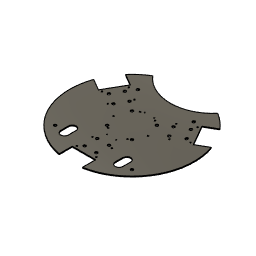
Plate_Mid+Desenho (Autodesk Fusion 360 archive; units mm, degrees)
design "Plate_Mid"
Autodesk Fusion 360 part; units mm, degrees
sketch "Esboço1" plane through (0, 0, 0) normal (0, 0, 1) x (1, 0, 0)
  circle A0 centre (0, 0) radius 240
  line L0 (48, -48) -> (-48, -48)
  line L1 (-48, -48) -> (-48, 48)
  line L2 (-48, 48) -> (48, 48)
  line L3 (48, 48) -> (48, -48)
  line L4 (48, -48) -> (-48, 48) construction
  line L5 (-48, -48) -> (48, 48) construction
  circle A1 centre (-48, 48) radius 5
  circle A2 centre (-48, -48) radius 5
  circle A3 centre (48, 48) radius 5
  circle A4 centre (48, -48) radius 5
  line L6 (105, -110) -> (105, -170)
  line L7 (90, -125) -> (90, -155)
  line L8 (120, -125) -> (120, -155)
  arc A5 (120, -125) -> (90, -125) centre (105, -125) ccw
  arc A6 (90, -155) -> (120, -155) centre (105, -155) ccw
  circle A7 centre (148, -148) radius 5
  line L9 (-125, 204.878) -> (125, 204.878)
  circle A8 centre (0, 311.043) radius 164
  circle A9 centre (107.5, 130.5) radius 5
  line L10 (-40, 115) -> (40, 115)
  line L11 (-40, 115) -> (-40, 151.9958)
  line L12 (40, 115) -> (40, 151.9958)
  line L13 (0, 1.75) -> (0, 22.5)
  line L14 (-120, -125) -> (-120, -155)
  arc A10 (-90, -125) -> (-120, -125) centre (-105, -125) ccw
  line L15 (-90, -125) -> (-90, -155)
  arc A11 (-120, -155) -> (-90, -155) centre (-105, -155) ccw
  circle A12 centre (-148, -148) radius 5
  circle A13 centre (-107.5, 130.5) radius 5
  line L16 (-45, -185) -> (45, -185)
  line L17 (45, -185) -> (45, -240)
  line L18 (45, -240) -> (-45, -240)
  line L19 (-45, -240) -> (-45, -185)
  line L20 (0, -185) -> (0, -175)
  line L21 (-37.5, -175) -> (37.5, -175)
  circle A14 centre (-37.5, -175) radius 2.5
  circle A15 centre (37.5, -175) radius 2.5
  circle A16 centre (37.5, -115) radius 2.5
  circle A17 centre (37.5, -55) radius 2.5
  circle A18 centre (-37.5, -115) radius 2.5
  circle A19 centre (-37.5, -55) radius 2.5
  circle A20 centre (132.8044, 119.976) radius 2.5
  line L22 (230.3461, 81.0289) -> (182.7147, 53.5289)
  line L23 (182.7147, 53.5289) -> (137.7147, 131.4711)
  line L24 (137.7147, 131.4711) -> (185.3461, 158.9711)
  circle A21 centre (80.8429, 89.976) radius 2.5
  circle A22 centre (170.3044, 55.024) radius 2.5
  circle A23 centre (118.3429, 25.024) radius 2.5
  circle A24 centre (66.3814, -4.976) radius 2.5
  circle A25 centre (28.8814, 59.976) radius 2.5
  circle A26 centre (-170.3044, 55.024) radius 2.5
  line L25 (-185.3461, 158.9711) -> (-137.7147, 131.4711)
  line L26 (-137.7147, 131.4711) -> (-182.7147, 53.5289)
  line L27 (-182.7147, 53.5289) -> (-230.3461, 81.0289)
  circle A27 centre (-118.3429, 25.024) radius 2.5
  circle A28 centre (-132.8044, 119.976) radius 2.5
  circle A29 centre (-80.8429, 89.976) radius 2.5
  circle A30 centre (-28.8814, 59.976) radius 2.5
  circle A31 centre (-66.3814, -4.976) radius 2.5
  line L28 (0, -185) -> (0, -160)
  line L29 (-22.5, -160) -> (22.5, -160)
  circle A32 centre (-22.5, -160) radius 5
  circle A33 centre (22.5, -160) radius 5
  circle A34 centre (-22.5, -111) radius 5
  circle A35 centre (22.5, -111) radius 5
  circle A36 centre (149.8141, 60.5144) radius 5
  circle A37 centre (107.3788, 36.0144) radius 5
  circle A38 centre (84.8788, 74.9856) radius 5
  circle A39 centre (127.3141, 99.4856) radius 5
  circle A40 centre (-127.3141, 99.4856) radius 5
  circle A41 centre (-84.8788, 74.9856) radius 5
  circle A42 centre (-107.3788, 36.0144) radius 5
  circle A43 centre (-149.8141, 60.5144) radius 5
  line L30 (-17.902, -79) -> (18.098, -79)
  circle A44 centre (-17.902, -79) radius 1.75
  circle A45 centre (18.098, -79) radius 1.75
  line L31 (0, 311.043) -> (0, 115)
  circle A46 centre (-17.902, 67) radius 1.75
  circle A47 centre (18.098, 67) radius 1.75
  point P0 (105, -110)
  point P1 (0, 115)
  point P2 (0, -240)
  point P3 (-45, -235.7435)
  point P4 (-181.6599, 156.8429)
  point P5 (181.6599, 156.8429)
  point P6 (0.098, -79)
  dimension "d1" = 480
  dimension "d2" = 96
  dimension "d3" = 96
  dimension "d4" = 10
  dimension "d5" = 10
  dimension "d6" = 10
  dimension "d7" = 10
  dimension "d8" = 110
  dimension "d9" = 105
  dimension "d10" = 30
  dimension "d11" = 60
  dimension "d12" = 30
  dimension "d13" = 10
  dimension "d14" = 148
  dimension "d15" = 148
  dimension "d16" = 250
  dimension "d17" = 328
  dimension "d18" = 10
  dimension "d19" = 130.5
  dimension "d20" = 107.5
  dimension "d21" = 115
  dimension "d22" = 80
  dimension "d25" = 90
  dimension "d26" = 55
  dimension "d27" = 10
  dimension "d28" = 75
  dimension "d29" = 5
  dimension "d30" = 5
  dimension "d33" = 1
  dimension "d34" = 60
  dimension "d36" = 360
  dimension "d37" = 25
  dimension "d38" = 45
  dimension "d39" = 10
  dimension "d40" = 10
  dimension "d43" = 0
  dimension "d44" = 49
  dimension "d45" = 36
  dimension "d46" = 3.5
  dimension "d47" = 3.5
  dimension "d51" = 0
  dimension "d52" = 146
  dimension "d53" = 32
  constraint coincident A0.centre origin
  constraint horizontal L0
  constraint perpendicular L0 L1
  constraint parallel L0 L2
  constraint parallel L1 L3
  constraint coincident L4 A0.centre
  constraint coincident L5 A0.centre
  constraint coincident L1.end L2.start
  constraint coincident L0.end L1.start
  constraint coincident L2.end L3.start
  constraint coincident L0.start L3.end
  constraint coincident P0 A5
  constraint coincident P0 L6.start
  constraint vertical L6
  constraint coincident A5.centre L6
  constraint coincident L6.end A6
  constraint tangent L7 A6
  constraint parallel L6 L7
  constraint tangent L8 A6
  constraint parallel L6 L8
  constraint horizontal L9
  constraint coincident A0 L9.start
  constraint coincident A0 L9.end
  constraint coincident L9.start A8
  constraint coincident L9.end A8
  constraint horizontal L10
  constraint midpoint P1 L10
  constraint coincident A8 L11.end
  constraint perpendicular L10 L11
  constraint coincident A8 L12.end
  constraint perpendicular L10 L12
  constraint symmetric L7.start L13 A10.start
  constraint symmetric L7.end L13 L15.end
  constraint symmetric L8.start L13 L14.start
  constraint symmetric L8.end L13 L14.end
  constraint symmetric A5 L13 A10
  constraint symmetric A6 L13 A11
  constraint symmetric A7 L13 A12
  constraint symmetric A9 L13 A13
  constraint horizontal L16
  constraint vertical L17
  constraint horizontal L18
  constraint vertical L19
  constraint midpoint L18 P2
  constraint tangent A0 L18
  constraint coincident A0 P2
  constraint midpoint L16 L20.start
  constraint perpendicular L16 L20
  constraint horizontal L21
  constraint midpoint L20.end L21
  constraint coincident L21.start A14.centre
  constraint coincident L21.end A15.centre
  constraint coincident A0 P3
  constraint coincident L19 P3
  constraint coincident L25 P4
  constraint coincident A0 P4
  constraint coincident L24 P5
  constraint coincident A0 P5
  constraint perpendicular L21 L28
  constraint horizontal L29
  constraint midpoint L28.end L29
  constraint coincident L29.start A32.centre
  constraint coincident L29.end A33.centre
  constraint horizontal L30
  constraint coincident L30.start A44.centre
  constraint coincident L30.end A45.centre
  constraint coincident A8.centre L31.start
  constraint coincident P1 L31.end
  constraint vertical L31
  constraint midpoint L30 P6
  measures "d1" diameter of A0
  measures "d2" distance of L1.end L2.end
  measures "d3" distance of L0.end L1.end
  measures "d4" diameter of A1
  measures "d5" diameter of A2
  measures "d6" diameter of A3
  measures "d7" diameter of A4
  measures "d8" vertical distance of A0.centre P0
  measures "d9" horizontal distance of A0.centre P0
  measures "d10" diameter of A5
  measures "d11" distance of P0 L6.end
  measures "d12" diameter of A6
  measures "d13" diameter of A7
  measures "d14" vertical distance of A0.centre A7.centre
  measures "d15" horizontal distance of A0.centre A7.centre
  measures "d16" distance of L9.start L9.end
  measures "d17" diameter of A8
  measures "d18" diameter of A9
  measures "d19" vertical distance of A0.centre A9.centre
  measures "d20" horizontal distance of A0.centre A9.centre
  measures "d21" distance of A0.centre L31.end
  measures "d22" distance of L10.start L10.end
  measures "d25" distance of L16.start L16.end
  measures "d26" distance of L16.start L18.end
  measures "d27" distance of L20.start L20.end
  measures "d28" distance of L21.start L21.end
  measures "d29" diameter of A14
  measures "d30" diameter of A15
  measures "d37" distance of L20.start L28.end
  measures "d38" distance of L29.start L29.end
  measures "d39" diameter of A32
  measures "d40" diameter of A33
  measures "d45" distance of L30.start L30.end
  measures "d46" diameter of A44
  measures "d47" diameter of A45
  measures "d53" vertical distance of A34.centre P6
extrude "Extrusão1" add sketch "Esboço1" along normal blind 3 contours A0 A8 L10 L11 L12 L16 L17 L19 L22 L23 L24 L25 L26 L27 | A8 L10 L12 L31 | A8 L10 L11 L31 | L0 L1 L2 L3 A1 A2 A3 A4
equation "d12 = d10"
equation "d17 = ( 164 * 2 ) * 1 mm"
